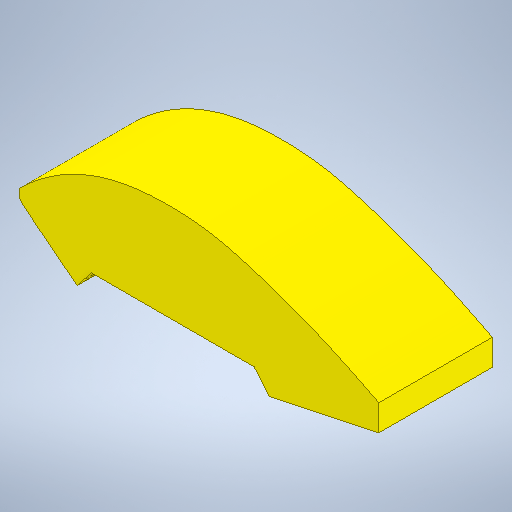
# Autodesk Inventor part: F-WheelPants
Saved by Autodesk Inventor 2025.3 (Build 293356000, 356)
## iProperties
Created: 2025-07-09
Part Number: F-WheelPants
Material: Generic
Document SubType Name: Modeling
Designer: steve
Density: 1 g/cm^3
Appearance: Default(1)
Author: steve
Autodesk Inventor part; units mm, degrees
ref_plane "YZ Plane" through (0, 0, 0) normal (1, 0, 0) x (0, 1, 0)
ref_plane "XZ Plane" through (0, 0, 0) normal (0, 1, 0) x (-1, 0, 0)
ref_plane "XY Plane" through (0, 0, 0) normal (0, 0, 1) x (1, 0, 0)
sketch "Sketch1" plane through (0, 0, 0) normal (0, 0, 1) x (1, 0, 0)
  line L0 (0, 0) -> (0, 11.7)
  line L1 (0, 11.7) -> (-17.808098, 20.803387) construction
  line L2 (-17.808098, 20.803387) -> (-17.808098, -4.366613) construction
  line L3 (-17.808098, 20.803387) -> (-36.228417, 28.593884) construction
  line L4 (-36.228417, 28.593884) -> (-36.228417, -7.036116) construction
  line L5 (-36.228417, 28.593884) -> (-55.195174, 34.939127) construction
  line L6 (-55.195174, 34.939127) -> (-55.195174, -9.670873) construction
  line L7 (-55.195174, 34.939127) -> (-74.374386, 40.609915) construction
  line L8 (-74.374386, 40.609915) -> (-74.374386, -1.710085) construction
  line L9 (-74.374386, 40.609915) -> (-94.331917, 41.912589) construction
  line L10 (-94.331917, 41.912589) -> (-94.331917, -2.507411) construction
  line L11 (-94.331917, 41.912589) -> (-114.289448, 40.609915) construction
  line L12 (-114.289448, 40.609915) -> (-114.289448, -1.700085) construction
  line L13 (-114.289448, 40.609915) -> (-133.46866, 34.939127) construction
  line L14 (-133.46866, 34.939127) -> (-133.46866, -4.930873) construction
  line L15 (-133.46866, 34.939127) -> (-150.648076, 24.698635) construction
  line L16 (-150.648076, 24.698635) -> (-150.648076, 8.628635) construction
  line L17 (-150.648076, 24.698635) -> (-161.411826, 14.681933) construction
  line L18 (-161.411826, 14.681933) -> (-161.411826, 9.681933)
  line L19 (-133.212221, -2.32016) -> (-56.045584, -2.32016) construction
  line L20 (-56.045584, -2.32016) -> (-49.29029, -10.449754) construction
  line L21 (-49.29029, -10.449754) -> (0, 0) construction
  line L22 (0, 11.7) -> (-17.808098, 20.803387) construction
  line L23 (-17.808098, 20.803387) -> (-36.228417, 28.593884) construction
  line L24 (-36.228417, 28.593884) -> (-55.195174, 34.939127) construction
  line L25 (-55.195174, 34.939127) -> (-74.374386, 40.609915) construction
  line L26 (-74.374386, 40.609915) -> (-94.331917, 41.912589) construction
  line L27 (-94.331917, 41.912589) -> (-114.289448, 40.609915) construction
  line L28 (-114.289448, 40.609915) -> (-133.46866, 34.939127) construction
  line L29 (-133.46866, 34.939127) -> (-150.648076, 24.698635) construction
  line L30 (-150.648076, 24.698635) -> (-161.411826, 14.681933) construction
  line L31 (-161.411826, 14.681933) -> (-163.905372, 12.361449) construction
  line L32 (-163.905372, 12.361449) -> (-161.411826, 9.681933) construction
  line L33 (-161.411826, 9.681933) -> (-146.00556, -2.32016) construction
  spline S0 degree 4 poles (0, 11.7) (-17.808098, 20.803387) (-36.228417, 28.593884) (-55.195174, 34.939127) (-74.374386, 40.609915) (-94.331917, 41.912589) (-114.289448, 40.609915) (-133.46866, 34.939127) (-150.648076, 24.698635) (-161.411826, 14.681933) (-163.905372, 12.361449) (-161.411826, 9.681933) (-146.00556, -2.32016) knots 1 1 1 1 1 2 3 4 5 6 7 8 9 10 10 10 10 10
  line L34 (-161.411826, 9.681933) -> (-135.570155, -10.449754)
  line L35 (-135.570155, -10.449754) -> (-129.236878, -2.32016)
  line L36 (-129.236878, -2.32016) -> (-56.045584, -2.32016)
  line L37 (-56.045584, -2.32016) -> (-49.29029, -10.449754)
  line L38 (-49.29029, -10.449754) -> (0, 0)
  point P0 (-161.411826, 14.46336)
  point P1 (-161.411826, 10.343905)
  dimension "d0" = 11.7
  dimension "d1" = 20
  dimension "d2" = 25.17
  dimension "d3" = 20
  dimension "d4" = 35.63
  dimension "d5" = 20
  dimension "d6" = 44.61
  dimension "d7" = 20
  dimension "d8" = 42.32
  dimension "d9" = 20
  dimension "d10" = 44.42
  dimension "d11" = 20
  dimension "d12" = 42.31
  dimension "d13" = 20
  dimension "d14" = 39.87
  dimension "d15" = 20
  dimension "d16" = 16.07
  dimension "d18" = 5
  constraints: 54 end point, 11 coincident, 11 collinear, 10 vertical, 3 perpendicular, 3 point on line, 3 other
  measures "d0" distance of L0.start L0.end
  measures "d1" distance of L0.end L1.end
  measures "d2" distance of L1.end L2.end
  measures "d3" distance of L1.end L3.end
  measures "d4" distance of L3.end L4.end
  measures "d5" distance of L3.end L5.end
  measures "d6" distance of L5.end L6.end
  measures "d7" distance of L5.end L7.end
  measures "d8" distance of L7.end L8.end
  measures "d9" distance of L7.end L9.end
  measures "d10" distance of L9.end L10.end
  measures "d11" distance of L9.end L11.end
  measures "d12" distance of L11.end L12.end
  measures "d13" distance of L11.end L13.end
  measures "d14" distance of L13.end L14.end
  measures "d15" distance of L13.end L15.end
  measures "d16" distance of L15.end L16.end
  measures "d18" distance of L18.end L17.end
sketch "Sketch1 outline for Extrusion1" plane through (0, 0, 0) normal (0, 0, 1) x (1, 0, 0)
  line L0 (0, 0) -> (0, 11.7)
  line L1 (-49.29029, -10.449754) -> (0, 0)
  line L2 (-56.045584, -2.32016) -> (-49.29029, -10.449754)
  line L3 (-129.236878, -2.32016) -> (-56.045584, -2.32016)
  line L4 (-135.570155, -10.449754) -> (-129.236878, -2.32016)
  line L5 (-146.00556, -2.32016) -> (-135.570155, -10.449754)
  spline S0 degree 4 poles (-161.411826, 10.343905) (-160.249352, 9.082913) (-158.012669, 7.129136) (-153.839823, 3.783043) (-146.00556, -2.32016) knots 0 0 0 0 0 1 1 1 1 1
  line L6 (-161.411826, 14.46336) -> (-161.411826, 10.343905)
  spline S1 degree 4 poles (0, 11.7) (-17.808098, 20.803387) (-36.228417, 28.593884) (-55.195174, 34.939127) (-74.374386, 40.609915) (-94.331917, 41.912589) (-114.289448, 40.609915) (-133.46866, 34.939127) (-149.653381, 25.291563) (-157.445761, 18.34705) (-160.515633, 15.512952) (-161.411826, 14.46336) knots 0 0 0 0 0 0.12872666 0.25745332 0.38617998 0.51490664 0.6436333 0.77235995 0.90108661 1 1 1 1 1
extrude "Extrusion1" add sketch "Sketch1 outline for Extrusion1" along normal mid plane 51
sketch "Sketch2" plane through (-129.236878, -2.32016, 25.5) normal (0, -1, 0) x (1, 0, 0)
  line L0 (73.191293, -51) -> (73.191293, 0)
  line L1 (0, 0) -> (73.191293, 0)
  line L2 (0, -51) -> (0, 0)
  line L3 (73.191293, -51) -> (0, -51)
  line L4 (6.095647, -25.5) -> (6.095647, -14)
  line L5 (6.095647, -14) -> (67.095647, -14)
  line L6 (67.095647, -14) -> (67.095647, -37)
  line L7 (67.095647, -37) -> (6.095647, -37)
  line L8 (6.095647, -37) -> (6.095647, -25.5)
  point P0 (129.236878, -25.5)
  point P1 (36.595647, -25.5)
  dimension "d24" = 30.5
  dimension "d25" = 11.5
  dimension "d26" = 61
  dimension "d27" = 23
  constraints: 10 end point, 4 perpendicular, 1 point on line
  measures "d24" distance of point (36.596, -25.5) L4.start
  measures "d25" distance of L4.start L4.end
  measures "d26" distance of L4.end L5.end
  measures "d27" distance of L5.end L6.end
extrude "Extrusion2" cut sketch "Sketch2" against normal blind 30 contours L4 L5 L6 L7 L8
body "Solid1"
